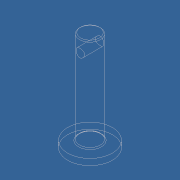
# Autodesk Inventor part: EIXO DAS ENGRENAGENS(11)
Saved by Autodesk Inventor 2012 SP1 (Build 160190100, 190)
## iProperties
Created: 2012-07-24
Part Number: EIXO DAS ENGRENAGENS(11)
Material: Carbon Steel
Document SubType Name: Modeling
Designer: bruno.silveira
Mass: 137.146 g
Surface Area: 39.6822 cm^2
Volume: 17.4264 cm^3
Density: 7.87 g/cm^3
Author: bruno.silveira
Autodesk Inventor part; units mm, degrees
ref_plane "YZ Plane" through (0, 0, 0) normal (1, 0, 0) x (0, 1, 0)
ref_plane "XZ Plane" through (0, 0, 0) normal (0, 1, 0) x (-1, 0, 0)
ref_plane "XY Plane" through (0, 0, 0) normal (0, 0, 1) x (1, 0, 0)
sketch "Sketch1" plane through (0, 0, 0) normal (0, 0, 1) x (1, 0, 0)
  circle A0 centre (0, 0) radius 10.75
  dimension "d0" = 21.5
  constraints: 1 centre point, 1 coincident
  measures "d0" diameter of A0
extrude "Extrusion1" add sketch "Sketch1" along normal blind 48
sketch "Sketch2" plane through (0, 0, 48) normal (0, 0, 1) x (1, 0, 0)
  circle A0 centre (0, 0) radius 10.75 projected
  circle A1 centre (0, 0) radius 5
  dimension "d3" = 10
  constraints: 1 centre point, 1 coincident
  measures "d3" diameter of A1
extrude "Extrusion2" cut sketch "Sketch2" against normal blind 45
chamfer "Chamfer1" distance 0.5 angle 45 1 edges at (-5, 0, 48)
fillet "Fillet1" radius 0.5 1 edges at (-5, 0, 3)
sketch "Sketch3" plane through (0, 0, 0) normal (0, 1, 0) x (-1, 0, 0)
  line L0 (-4.5, 48) -> (4.5, 48) projected
  line L1 (5, 47.5) -> (-5, 47.5) projected
  line L2 (-5, 3.5) -> (5, 3.5) projected
  circle A0 centre (0, 42) radius 2
  point P0 (0, 0)
  dimension "d10" = 4
  dimension "d11" = 6
  constraints: 1 centre point
  measures "d10" diameter of A0
  measures "d11" distance from line of L0 A0.centre
extrude "Extrusion3" cut sketch "Sketch3" along normal mid plane 15
body "Solid1"
